Support Camera (Autodesk Fusion 360 design; units mm, degrees)
Autodesk Fusion 360 part; units mm, degrees
note: some values were not read from the file. Set by a fixed rule: which sketch regions a step uses.
sketch "Support Cam" plane through (0, 0, 0) normal (0, 0, 1) x (1, 0, 0)
  line L0 (-198.7446, -257.0866) -> (-125.8054, -257.0866)
  line L1 (-125.8054, -257.0866) -> (-125.8054, -260.9951)
  line L2 (-125.8054, -260.9951) -> (-120.4545, -260.9951)
  line L3 (-120.4545, -260.9951) -> (-120.4545, -255.1026)
  line L4 (-120.4545, -255.1026) -> (-80.9396, -255.1026)
  line L5 (-80.9396, -255.1026) -> (-80.9396, -260.7322)
  line L6 (-80.9396, -260.7322) -> (-75.0474, -260.7322)
  line L7 (-75.0474, -260.7322) -> (-75.0474, -257.0778)
  line L8 (-75.0474, -257.0778) -> (-62.9514, -257.0778)
  line L9 (-62.9514, -257.0778) -> (-62.9514, -254.5567)
  line L10 (-62.9514, -254.5567) -> (-58.1923, -250.6191)
  line L11 (-58.1923, -250.6191) -> (-53.9714, -250.6191)
  line L12 (-53.9714, -250.6191) -> (-53.9714, -241.0645)
  line L13 (-53.9714, -241.0645) -> (-58.456, -236.613)
  line L14 (-58.456, -236.613) -> (-58.456, -217.7866)
  line L15 (-58.456, -217.7866) -> (-53.9714, -217.7866)
  line L16 (-53.9714, -217.7866) -> (-53.9714, -193.3927)
  line L17 (-53.9714, -193.3927) -> (-60.1213, -193.3927)
  line L18 (-60.1213, -193.3927) -> (-60.1213, -191.7009)
  line L19 (-60.1213, -191.7009) -> (-53.9714, -191.7009)
  line L20 (-53.9714, -191.7009) -> (-53.9714, -181.6027)
  line L21 (-53.9714, -181.6027) -> (-199.5171, -181.6027)
  line L22 (-199.5171, -181.6027) -> (-199.5171, -214.5082)
  line L23 (-199.5171, -214.5082) -> (-202.4466, -214.5082)
  line L24 (-202.4466, -214.5082) -> (-202.4466, -235.0144)
  line L25 (-202.4466, -235.0144) -> (-208.3055, -241.7413)
  line L26 (-208.3055, -241.7413) -> (-208.3055, -250.4212)
  line L27 (-208.3055, -250.4212) -> (-202.4466, -250.4212)
  line L28 (-202.4466, -250.4212) -> (-198.7446, -257.0866)
  line L29 (-202.4466, -214.5082) -> (-178.9466, -214.5082) construction
  line L30 (-178.9466, -214.5082) -> (-178.9466, -253.5082) construction
  line L31 (-178.9466, -253.5082) -> (-202.4466, -253.5082) construction
  line L32 (-202.4466, -253.5082) -> (-202.4466, -214.5082) construction
  line L33 (-83.4128, -214.476) -> (-59.9128, -214.476) construction
  line L34 (-59.9128, -214.476) -> (-59.9128, -253.476) construction
  line L35 (-59.9128, -253.476) -> (-83.4128, -253.476) construction
  line L36 (-83.4128, -253.476) -> (-83.4128, -214.476) construction
  line L37 (-176.7676, -200.3683) -> (-154.7676, -200.3683) construction
  line L38 (-154.7676, -200.3683) -> (-154.7676, -185.3683) construction
  line L39 (-154.7676, -185.3683) -> (-176.7676, -185.3683) construction
  line L40 (-176.7676, -185.3683) -> (-176.7676, -200.3683) construction
  line L41 (-107.7676, -185.3683) -> (-107.7676, -200.3683) construction
  line L42 (-107.7676, -200.3683) -> (-85.7676, -200.3683) construction
  line L43 (-85.7676, -200.3683) -> (-85.7676, -185.3683) construction
  line L44 (-85.7676, -185.3683) -> (-107.7676, -185.3683) construction
  line L45 (-190.6966, -253.5082) -> (-190.6966, -214.5082) construction
  circle A0 centre (-190.6966, -238.5082) radius 1.1
  circle A1 centre (-190.6966, -224.5082) radius 1.1
  line L46 (-71.6628, -253.476) -> (-71.6628, -214.476) construction
  circle A2 centre (-71.6628, -238.476) radius 1.1
  circle A3 centre (-71.6628, -224.476) radius 1.1
  line L47 (-176.7676, -192.8683) -> (-154.7676, -192.8683) construction
  line L48 (-107.7676, -192.8683) -> (-85.7676, -192.8683) construction
  circle A4 centre (-171.7676, -192.8683) radius 1.1
  circle A5 centre (-159.7676, -192.8683) radius 1.1
  circle A6 centre (-102.7676, -192.8683) radius 1.1
  circle A7 centre (-90.7676, -192.8683) radius 1.1
  line L49 (-141.6035, -233.9087) -> (-141.6035, -212.4087) construction
  line L50 (-141.6035, -212.4087) -> (-113.6035, -212.4087) construction
  line L51 (-113.6035, -212.4087) -> (-113.6035, -233.9087) construction
  line L52 (-113.6035, -233.9087) -> (-141.6035, -233.9087) construction
  line L53 (-118.6035, -228.9087) -> (-136.6035, -228.9087) construction
  line L54 (-136.6035, -228.9087) -> (-136.6035, -217.4087) construction
  line L55 (-136.6035, -217.4087) -> (-118.6035, -217.4087) construction
  line L56 (-118.6035, -217.4087) -> (-118.6035, -228.9087) construction
  circle A8 centre (-136.6035, -228.9087) radius 1.1
  circle A9 centre (-118.6035, -228.9087) radius 1.1
  circle A10 centre (-118.6035, -217.4087) radius 1.1
  circle A11 centre (-136.6035, -217.4087) radius 1.1
  circle A12 centre (-188.7259, -245.8252) radius 2.6
  circle A13 centre (-188.7259, -190.3252) radius 2.6
  circle A14 centre (-69.2259, -190.3252) radius 2.6
  circle A15 centre (-69.2259, -245.8252) radius 2.6
  line L57 (-154.7676, -192.8683) -> (-107.7676, -192.8683) construction
  line L58 (-141.2676, -197.8683) -> (-121.2676, -197.8683)
  arc A16 (-121.2676, -197.8683) -> (-121.2676, -187.8683) centre (-121.2676, -192.8683) ccw
  line L59 (-121.2676, -187.8683) -> (-141.2676, -187.8683)
  arc A17 (-141.2676, -187.8683) -> (-141.2676, -197.8683) centre (-141.2676, -192.8683) ccw
  line L60 (-141.2676, -192.8683) -> (-121.2676, -192.8683) construction
  line L61 (-183.7259, -250.8252) -> (-74.2259, -250.8252) construction
  line L62 (-74.2259, -250.8252) -> (-74.2259, -185.3252) construction
  line L63 (-74.2259, -185.3252) -> (-183.7259, -185.3252) construction
  line L64 (-183.7259, -185.3252) -> (-183.7259, -250.8252) construction
  line L65 (-183.5759, -185.4752) -> (-183.5759, -250.6752)
  line L66 (-183.5759, -250.6752) -> (-74.3759, -250.6752)
  line L67 (-74.3759, -250.6752) -> (-74.3759, -185.4752)
  line L68 (-74.3759, -185.4752) -> (-183.5759, -185.4752)
  circle A18 centre (-136.6035, -217.4087) radius 2.5
  circle A19 centre (-118.6035, -217.4087) radius 2.5
  circle A20 centre (-136.6035, -228.9087) radius 2.5
  circle A21 centre (-118.6035, -228.9087) radius 2.5
  circle A22 centre (-71.6628, -224.476) radius 2.5
  circle A23 centre (-71.6628, -238.476) radius 2.5
  circle A24 centre (-190.6966, -224.5082) radius 2.5
  circle A25 centre (-190.6966, -238.5082) radius 2.5
  circle A26 centre (-171.7676, -192.8683) radius 2.5
  circle A27 centre (-159.7676, -192.8683) radius 2.5
  circle A28 centre (-102.7676, -192.8683) radius 2.5
  circle A29 centre (-90.7676, -192.8683) radius 2.5
  line L69 (-176.7676, -243.3252) -> (-154.7676, -243.3252) construction
  circle A30 centre (-171.7676, -243.3252) radius 1.1
  circle A31 centre (-159.7676, -243.3252) radius 1.1
  circle A32 centre (-171.7676, -243.3252) radius 2.5
  circle A33 centre (-159.7676, -243.3252) radius 2.5
  circle A34 centre (-90.7676, -243.3252) radius 2.5
  circle A35 centre (-102.7676, -243.3252) radius 2.5
  circle A36 centre (-90.7676, -243.3252) radius 1.1
  line L70 (-107.7676, -243.3252) -> (-85.7676, -243.3252) construction
  circle A37 centre (-102.7676, -243.3252) radius 1.1
  point P0 (-188.7259, -245.8252)
  point P1 (-188.7259, -190.3252)
  point P2 (-69.2259, -190.3252)
  point P3 (-69.2259, -245.8252)
  point P4 (-131.2676, -192.8683)
  point P5 (-183.7259, -185.3252)
  point P6 (-183.7259, -250.8252)
  point P7 (-74.2259, -250.8252)
  point P8 (-74.2259, -185.3252)
  dimension "d165" = 23.5
  dimension "d166" = 39
  dimension "d167" = 23.5
  dimension "d168" = 39
  dimension "d169" = 22
  dimension "d170" = 15
  dimension "d171" = 22
  dimension "d172" = 15
  dimension "d175" = 2.2
  dimension "d176" = 2.2
  dimension "d177" = 10
  dimension "d178" = 15
  dimension "d179" = 2.2
  dimension "d180" = 2.2
  dimension "d181" = 10
  dimension "d182" = 15
  dimension "d183" = 2.2
  dimension "d184" = 5
  dimension "d185" = 2.2
  dimension "d186" = 2.2
  dimension "d187" = 2.2
  dimension "d188" = 5
  dimension "d189" = 5
  dimension "d190" = 5
  dimension "d195" = 21.5
  dimension "d196" = 28
  dimension "d197" = 5
  dimension "d198" = 2.2
  dimension "d199" = 2.2
  dimension "d200" = 2.2
  dimension "d201" = 2.2
  dimension "d204" = 5.2
  dimension "d205" = 5.2
  dimension "d206" = 5.2
  dimension "d207" = 5.2
  dimension "d210" = 10
  dimension "d248" = -0.15
  dimension "d253" = 5
  dimension "d254" = 5
  dimension "d255" = 5
  dimension "d256" = 5
  dimension "d259" = 5
  dimension "d260" = 5
  dimension "d261" = 5
  dimension "d262" = 5
  dimension "d265" = 5
  dimension "d266" = 5
  dimension "d267" = 5
  dimension "d268" = 5
  dimension "d365" = 2.2
  dimension "d366" = 5
  dimension "d367" = 2.2
  dimension "d368" = 2.2
  dimension "d369" = 2.2
  dimension "d370" = 5
  dimension "d371" = 5
  dimension "d372" = 5
  dimension "d373" = 5
  dimension "d374" = 5
  dimension "d375" = 5
  dimension "d376" = 5
  dimension "d377" = 7.5
  dimension "d378" = 7.5
  constraint horizontal L0
  constraint perpendicular L0 L1
  constraint perpendicular L1 L2
  constraint perpendicular L2 L3
  constraint perpendicular L3 L4
  constraint perpendicular L4 L5
  constraint perpendicular L3 L6
  constraint perpendicular L6 L7
  constraint perpendicular L7 L8
  constraint perpendicular L8 L9
  constraint perpendicular L9 L11
  constraint perpendicular L11 L12
  constraint perpendicular L11 L14
  constraint perpendicular L14 L15
  constraint perpendicular L15 L16
  constraint perpendicular L16 L17
  constraint perpendicular L17 L18
  constraint perpendicular L18 L19
  constraint perpendicular L19 L20
  constraint perpendicular L3 L21
  constraint perpendicular L21 L22
  constraint perpendicular L22 L23
  constraint perpendicular L23 L24
  constraint parallel L24 L26
  constraint perpendicular L26 L27
  constraint horizontal L29
  constraint vertical L30
  constraint horizontal L31
  constraint vertical L32
  constraint horizontal L33
  constraint vertical L34
  constraint horizontal L35
  constraint vertical L36
  constraint horizontal L37
  constraint vertical L38
  constraint horizontal L39
  constraint vertical L40
  constraint horizontal L42
  constraint vertical L43
  constraint horizontal L44
  constraint vertical L41
  constraint midpoint L31 L45.start
  constraint midpoint L29 L45.end
  constraint coincident L45 A0.centre
  constraint coincident L45 A1.centre
  constraint midpoint L35 L46.start
  constraint midpoint L33 L46.end
  constraint coincident L46 A2.centre
  constraint coincident L46 A3.centre
  constraint midpoint L40 L47.start
  constraint midpoint L38 L47.end
  constraint midpoint L41 L48.start
  constraint midpoint L43 L48.end
  constraint coincident L47 A4.centre
  constraint coincident L47 A5.centre
  constraint coincident L48 A6.centre
  constraint coincident L48 A7.centre
  constraint vertical L49
  constraint perpendicular L49 L50
  constraint perpendicular L50 L51
  constraint perpendicular L51 L52
  constraint coincident L53.end L54.start
  constraint coincident L53.start L56.end
  constraint coincident L55.end L56.start
  constraint coincident L54.end L55.start
  constraint coincident P0 A12.centre
  constraint coincident P1 A13.centre
  constraint coincident P2 A14.centre
  constraint coincident P3 A15.centre
  constraint perpendicular L41 L57
  constraint tangent L58 A16
  constraint tangent A16 L59
  constraint parallel L58 L59
  constraint tangent L59 A17
  constraint tangent L58 A17
  constraint perpendicular L30 L60
  constraint midpoint L57 P4
  constraint midpoint L60 P4
  constraint horizontal L61
  constraint vertical L62
  constraint horizontal L63
  constraint vertical L64
  constraint coincident P8 L62.end
  constraint coincident P6 L61.start
  constraint concentric A11 A18
  constraint concentric A10 A19
  constraint concentric A8 A20
  constraint concentric A9 A21
  constraint concentric A3 A22
  constraint concentric A2 A23
  constraint concentric A1 A24
  constraint concentric A0 A25
  constraint concentric A4 A26
  constraint concentric A5 A27
  constraint concentric A6 A28
  constraint concentric A7 A29
  constraint coincident A30.centre L69
  constraint coincident A31.centre L69
  constraint coincident A35.centre L70
  constraint coincident A34.centre L70
  constraint concentric A30 A32
  constraint concentric A31 A33
  constraint concentric A35 A37
  constraint concentric A34 A36
  measures "d165" distance of L23.end L29.end
  measures "d166" distance of L23.end L31.end
  measures "d167" distance of L33.start L33.end
  measures "d168" distance of L33.start L35.end
  measures "d169" distance of L37.start L37.end
  measures "d170" distance of L37.start L39.end
  measures "d171" distance of L42.end L41.end
  measures "d172" distance of L41.start L41.end
  measures "d175" diameter of A0
  measures "d176" diameter of A1
  measures "d177" distance of L45.end A1.centre
  measures "d178" distance of L31 A0.centre
  measures "d179" diameter of A2
  measures "d180" diameter of A3
  measures "d181" distance of L46.end A3.centre
  measures "d182" distance of L46.start A2.centre
  measures "d183" diameter of A4
  measures "d184" distance of L47.start A4.centre
  measures "d185" diameter of A5
  measures "d186" diameter of A6
  measures "d187" diameter of A7
  measures "d188" distance of L48.start A6.centre
  measures "d189" distance of L48.end A7.centre
  measures "d190" distance of L47.end A5.centre
  measures "d195" distance of L49.start L49.end
  measures "d196" distance of L49.start L51.end
  measures "d198" diameter of A8
  measures "d199" diameter of A9
  measures "d200" diameter of A10
  measures "d201" diameter of A11
  measures "d204" diameter of A12
  measures "d205" diameter of A13
  measures "d206" diameter of A14
  measures "d207" diameter of A15
  measures "d210" diameter of A16
  measures "d253" diameter of A18
  measures "d254" diameter of A19
  measures "d255" diameter of A20
  measures "d256" diameter of A21
  measures "d259" diameter of A22
  measures "d260" diameter of A23
  measures "d261" diameter of A24
  measures "d262" diameter of A25
  measures "d265" diameter of A26
  measures "d266" diameter of A27
  measures "d267" diameter of A28
  measures "d268" diameter of A29
  measures "d365" diameter of A30
  measures "d366" distance of A30.centre L69.start
  measures "d367" diameter of A31
  measures "d368" diameter of A37
  measures "d369" diameter of A36
  measures "d370" distance of A35.centre L70.start
  measures "d371" distance of L70.end A34.centre
  measures "d372" distance of L69.end A31.centre
  measures "d373" diameter of A32
  measures "d374" diameter of A33
  measures "d375" diameter of A35
  measures "d376" diameter of A34
  measures "d377" distance of L61 L70.start
  measures "d378" distance of L61 L69.end
extrude "Extrude9" add sketch "Support Cam" against normal blind 7 contours L0 L1 L2 L3 L4 L5 L6 L7 L8 L9 L10 L11 L12 L13 L14 L15 L16 L17 L18 L19 L20 L21 L22 L23 L24 L25 L26 L27 L28 | A12 | A13 | A14 | A15 | L65 L66 L67 L68 | A18 | A19 | A20 | A21 | A22 | A23 | A24 | A25 | A26 | A27 | A28 | A29 | A32 | A33 | A34 | A35
extrude "Extrude15" add sketch "Support Cam" along normal blind 2 contours L65 L66 L67 L68
extrude "Extrude16" cut sketch "Support Cam" against normal blind 3.1 contours A12 | A13 | A14 | A15
extrude "Extrude18" cut sketch "Support Cam" against normal blind 3.5 contours A18 | A19 | A20 | A21 | A22 | A23 | A24 | A25 | A26 | A27 | A28 | A29 | A32 | A33 | A34 | A35
equation "d175 = Trous_Vis_diam2"
equation "d176 = Trous_Vis_diam2"
equation "d179 = Trous_Vis_diam2"
equation "d180 = Trous_Vis_diam2"
equation "d183 = Trous_Vis_diam2"
equation "d185 = Trous_Vis_diam2"
equation "d186 = Trous_Vis_diam2"
equation "d187 = Trous_Vis_diam2"
equation "d198 = Trous_Vis_diam2"
equation "d199 = Trous_Vis_diam2"
equation "d200 = Trous_Vis_diam2"
equation "d201 = Trous_Vis_diam2"
equation "d365 = Trous_Vis_diam2"
equation "d367 = Trous_Vis_diam2"
equation "d368 = Trous_Vis_diam2"
equation "d369 = Trous_Vis_diam2"
equation "Trous_Vis_diam2 = 2.2 mm"
named bodies: "Support Cam"
